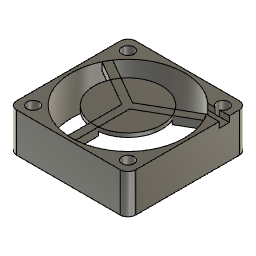
fan-frame-3010 (Autodesk Fusion 360 design; units mm, degrees)
Autodesk Fusion 360 part; units mm, degrees
sketch "Frame" plane through (0, 0, 0) normal (0, 0, 1) x (1, 0, 0)
  line L0 (13.2, -15.2) -> (-13.2, -15.2)
  line L1 (-15.2, -13.2) -> (-15.2, 13.2)
  line L2 (-13.2, 15.2) -> (13.2, 15.2)
  line L3 (15.2, 13.2) -> (15.2, -13.2)
  circle A0 centre (0, 0) radius 14.4
  arc A1 (13.2, -15.2) -> (15.2, -13.2) centre (13.2, -13.2) ccw
  arc A2 (-15.2, -13.2) -> (-13.2, -15.2) centre (-13.2, -13.2) ccw
  arc A3 (-13.2, 15.2) -> (-15.2, 13.2) centre (-13.2, 13.2) ccw
  arc A4 (15.2, 13.2) -> (13.2, 15.2) centre (13.2, 13.2) ccw
  circle A5 centre (-12.1, 12.1) radius 1.55
  line L4 (0, -20) -> (0, 21.5907) construction
  line L5 (25, 0) -> (-35, 0) construction
  circle A6 centre (12.1, 12.1) radius 1.55
  circle A7 centre (-12.1, -12.1) radius 1.55
  circle A8 centre (12.1, -12.1) radius 1.55
  dimension "d1" = 30.4
  dimension "d2" = 30.4
  dimension "d3" = 15.2
  dimension "d4" = 15.2
  dimension "d5" = 28.8
  dimension "d6" = 2
  dimension "d7" = 3.1
  dimension "d8" = 3.1
  dimension "d9" = 3.1
  constraint horizontal L0
  constraint vertical L1
  constraint horizontal L2
  constraint vertical L3
  constraint coincident A0.centre origin
  constraint tangent L0 A1
  constraint tangent L3 A1
  constraint tangent L0 A2
  constraint tangent L1 A2
  constraint equal A1 A2
  constraint tangent L1 A3
  constraint tangent L2 A3
  constraint equal A1 A3
  constraint tangent L2 A4
  constraint tangent L3 A4
  constraint equal A1 A4
  constraint vertical L4
  constraint coincident A0.centre L4
  constraint horizontal L5
  constraint coincident A0.centre L5
  constraint symmetric A5 L4 A6
  constraint symmetric A5 L5 A7
  constraint symmetric L5 A6 A8
  measures "d1" distance of L0 L2
  measures "d2" distance of L1 L3
  measures "d3" distance of A0.centre L0
  measures "d4" distance of A0.centre L1
  measures "d5" diameter of A0
  measures "d6" radius of A1
  measures "d7" diameter of A5
  measures "d8" distance of L1 A5.centre
  measures "d9" distance of L2 A5.centre
extrude "Extrude1" add sketch "Frame" along normal blind 10 makes body 1
sketch "Fan Attacher" plane through (0, 0, 10) normal (0, 0, 1) x (-1, 0, 0)
  circle A0 centre (-12.1, -12.1) radius 1.55
  circle A1 centre (-12.1, 12.1) radius 1.55
  circle A2 centre (0, 0) radius 14.4
  circle A3 centre (12.1, 12.1) radius 1.55
  circle A4 centre (12.1, -12.1) radius 1.55
  arc A5 (-13.2, 15.2) -> (-15.2, 13.2) centre (-13.2, 13.2) ccw
  line L0 (-15.2, 13.2) -> (-15.2, -13.2)
  arc A6 (-15.2, -13.2) -> (-13.2, -15.2) centre (-13.2, -13.2) ccw
  line L1 (-13.2, -15.2) -> (13.2, -15.2)
  arc A7 (13.2, -15.2) -> (15.2, -13.2) centre (13.2, -13.2) ccw
  line L2 (15.2, -13.2) -> (15.2, 13.2)
  arc A8 (15.2, 13.2) -> (13.2, 15.2) centre (13.2, 13.2) ccw
  line L3 (13.2, 15.2) -> (-13.2, 15.2)
  line L4 (0, 14.4) -> (0, 0) construction
  line L5 (0, 0) -> (-12.4708, -7.2) construction
  line L6 (0, 0) -> (12.4708, -7.2) construction
  line L7 (-1, 14.4) -> (-1, 0.5774)
  line L8 (1, 14.4) -> (1, 0.5774)
  line L9 (-1, 0.5774) -> (-12.9708, -6.334)
  line L10 (0, -1.1547) -> (-11.9708, -8.066)
  line L11 (0, -1.1547) -> (11.9708, -8.066)
  line L12 (1, 0.5774) -> (12.9708, -6.334)
  circle A9 centre (0, 0) radius 14.4
  dimension "d12" = 120
  dimension "d13" = 120
  constraint coincident A2 L4.start
  constraint coincident A2.centre L4.end
  constraint perpendicular L3 L4
  constraint coincident A2 L5.end
  constraint coincident A2 L6.end
  constraint coincident L6.end A9
  measures "d12" angle of L4 L5
  measures "d13" angle of L5 L6
extrude "Extrude2" add sketch "Fan Attacher" against normal blind 2 separate body contours A2 L7 L8 L9 L10 L11 L12 A9 makes body 2
sketch "Sketch3" plane through (0, 0, 8) normal (0, 0, -1) x (1, 0, 0)
  line L0 (1, 0.5774) -> (1, 14.3652) construction
  arc A0 (1, 14.3652) -> (-1, 14.3652) centre (0, 0) ccw
  line L1 (-1, 14.3652) -> (-1, 0.5774) construction
  line L2 (-1, 0.5774) -> (-12.9407, -6.3166) construction
  arc A1 (-12.9407, -6.3166) -> (-11.9407, -8.0486) centre (0, 0) ccw
  line L3 (-11.9407, -8.0486) -> (0, -1.1547) construction
  line L4 (0, -1.1547) -> (11.9407, -8.0486) construction
  arc A2 (11.9407, -8.0486) -> (12.9407, -6.3166) centre (0, 0) ccw
  line L5 (12.9407, -6.3166) -> (1, 0.5774)
  circle A3 centre (0, 0) radius 8.6
  dimension "d22" = 17.2
  constraint coincident A0.centre A1.centre
  measures "d22" diameter of A3
extrude "Extrude3" add sketch "Sketch3" against normal up to surface (2 mm away) separate body makes body 3
sketch "Sketch4" plane through (0, 0, 8) normal (0, 0, -1) x (1, 0, 0)
  circle A0 centre (0, 0) radius 8.6
  circle A1 centre (0, 0) radius 8.6
  dimension "d26" = 17.2
  constraint coincident A0.centre A1.centre
  measures "d26" diameter of A1
extrude "Extrude4" cut sketch "Sketch4" against normal blind 1 bodies 2 3
sketch "Sketch5" plane through (0, 0, 10) normal (0, 0, 1) x (-1, 0, 0)
  line L0 (-1, 14.3652) -> (-1, 0.5774)
  line L1 (-1, 0.5774) -> (-12.9407, -6.3166)
  arc A0 (-12.9407, -6.3166) -> (-11.9407, -8.0486) centre (0, 0) ccw
  line L2 (-11.9407, -8.0486) -> (0, -1.1547)
  line L3 (0, -1.1547) -> (11.9407, -8.0486)
  arc A1 (11.9407, -8.0486) -> (12.9407, -6.3166) centre (0, 0) ccw
  line L4 (12.9407, -6.3166) -> (1, 0.5774)
  line L5 (1, 0.5774) -> (1, 14.3652)
  arc A2 (1, 14.3652) -> (-1, 14.3652) centre (0, 0) ccw
  circle A3 centre (0, 0) radius 14.4
  line L6 (-11.9407, -8.0486) -> (-16, -8.0486)
  line L7 (-9.6936, -10.6486) -> (-16, -10.6486)
  line L8 (-16, -8.0486) -> (-16, -10.6486)
  dimension "d29" = 2.6
  dimension "d30" = 16
  constraint coincident A0.centre A1.centre
  constraint coincident A0.end A3
  constraint coincident A0.end L2.start
  constraint horizontal L6
  constraint coincident A3 L7.start
  constraint parallel L6 L7
  constraint perpendicular L7 L8
  measures "d29" distance of L6 L7
  measures "d30" distance of A0.centre L8
extrude "Extrude5" cut sketch "Sketch5" against normal blind 1.5 contours A3 L6 L7 L8 bodies 1
equation "d3 = ( 30.4 / 2 ) * 1 mm"
